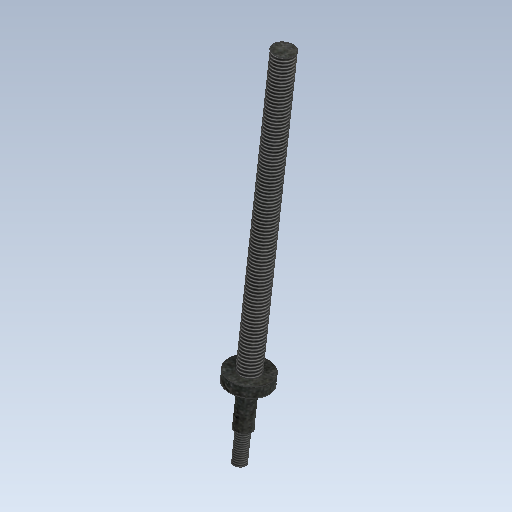
# Autodesk Inventor part: RA_csavar
Saved by Autodesk Inventor 2021.4 (Build 254397000, 397)
## iProperties
Created: 2023-11-22
Part Number: RA_csavar
Material: Steel
Document SubType Name: Modeling
Designer: ZenBook
Density: 7.85 g/cm^3
Appearance: Plate
Mass: 109.867 g
Surface Area: 61.2611 cm^2
Volume: 13.9958 cm^3
Author: ZenBook
Autodesk Inventor part; units mm, degrees
ref_plane "YZ Plane" through (0, 0, 0) normal (1, 0, 0) x (0, 1, 0)
ref_plane "XZ Plane" through (0, 0, 0) normal (0, 1, 0) x (-1, 0, 0)
derived "skeleton_1.ipt"
sketch "Sketch4" plane through (15.7936, 0, 654.9134) normal (0.6333709, 0.5, -0.5906279) x (-0.6819984, 0, -0.7313537)
  line L0 (0, 0) -> (145, 0) construction
  line L1 (45, 0) -> (45, -99)
  line L2 (45, -99) -> (39, -99)
sketch "Sketch6" plane through (25.3977, -85.7365, 592.6316) normal (0.7285714, -0.0871445, -0.6794038) x (-0.6819984, 0, -0.7313537)
  line L0 (6, 0) -> (0, 0) construction
  line L1 (0, 0) -> (0, 86.0639)
  line L2 (0, 86.0639) -> (-39, 86.0639)
  point P0 (-5, 86.0639)
  point P1 (4, 0)
  point P2 (-4, 0)
  point P3 (5, 86.0639)
ref_plane "Work Plane1" through (30.8829, 0, 587.5166) normal (-0.7285714, 0.0871445, 0.6794038) x (0.6819984, 0, 0.7313537)
sketch "Sketch5" plane through (30.8829, 0, 587.5166) normal (-0.7285714, 0.0871445, 0.6794038) x (0.6819984, 0, 0.7313537)
  line L0 (0, -180) -> (3, -180)
  line L1 (3, -180) -> (3, -165)
  line L2 (3, -165) -> (4, -165)
  line L3 (4, -165) -> (4, -145)
  line L4 (4, -145) -> (10, -145)
  line L5 (10, -145) -> (10, -140)
  line L6 (10, -140) -> (5, -140)
  line L7 (5, -140) -> (5, 0)
  line L8 (5, 0) -> (0, 0)
  line L9 (0, 0) -> (0, -180)
  line L10 (0, -86.0639) -> (0, 0) projected
  point P0 (-450.7445, 32.9493)
  point P1 (4, -86.0639)
  point P2 (5, 0)
  dimension "d14" = 5
  dimension "d15" = 20
  dimension "d16" = 15
  dimension "d18" = 20
  dimension "d19" = 6
  dimension "d20" = 180
  constraints: 20 end point, 9 perpendicular, 3 point on line, 1 collinear, 1 horizontal
  measures "d14" distance between parallel lines of L6 L4
  measures "d15" distance between parallel lines of L2 L4
  measures "d16" distance between parallel lines of L0 L2
  measures "d18" diameter of L5 L10
  measures "d19" diameter of L1 L10
  measures "d20" distance between parallel lines of L0 L8
revolve "Revolution2" add sketch "Sketch5" angle 360 about axis through (25.3977, -85.7365, 592.6316) along (0.0637335, 0.9961957, -0.0594324)
thread "Thread3" size "M10x1.5" class "6g" standard "ISO Metric profile" full length
thread "Thread4" size "M6x1" class "6g" standard "ISO Metric profile" full length
body "Solid1"
